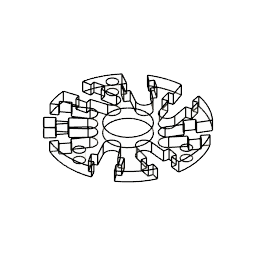
MidBearingMount-Mid_v21 (Autodesk Fusion 360 design; units mm, degrees)
Autodesk Fusion 360 part; units mm, degrees
other "Sketch1"
sketch "Sketch1" plane through (0, 0, 0) normal (0, 0, 1) x (1, 0, 0)
  circle A0 centre (0, 0) radius 20
  dimension "d1" = 40
  constraint coincident A0.centre origin
  measures "d1" diameter of A0
extrude "Extrude1" add sketch "Sketch1" along normal blind 3
sketch "sketch 220" plane through (0, 0, 0) normal (0, 0, 1) x (1, 0, 0)
  line L0 (55, -55) -> (-55, -55)
  line L1 (-55, -55) -> (-55, 55)
  line L2 (-55, 55) -> (55, 55)
  line L3 (55, 55) -> (55, -55)
  circle A0 centre (-27, 47) radius 3
  circle A1 centre (-1, 47) radius 3
  circle A2 centre (-47, -1) radius 3
  circle A3 centre (-47, -27) radius 3
  circle A4 centre (3.8268, 9.2388) radius 2.1
  line L4 (3.8268, 9.2388) -> (0, 0) construction
  circle A5 centre (-3.8268, 9.2388) radius 2.1
  circle A6 centre (-9.2388, 3.8268) radius 2.1
  circle A7 centre (-9.2388, -3.8268) radius 2.1
  circle A8 centre (-3.8268, -9.2388) radius 2.1
  circle A9 centre (3.8268, -9.2388) radius 2.1
  circle A10 centre (9.2388, -3.8268) radius 2.1
  circle A11 centre (9.2388, 3.8268) radius 2.1
  circle A12 centre (-47, -27) radius 3
  circle A13 centre (-47, -1) radius 3
  circle A14 centre (27, -47) radius 3
  circle A15 centre (1, -47) radius 3
  circle A16 centre (47, 27) radius 3
  circle A17 centre (47, 1) radius 3
  line L5 (3.8268, 9.2388) -> (-7.356, 51.4484) construction
  line L6 (-3.8267, 9.2387) -> (-39.1481, 32.3388) construction
  line L7 (-9.2241, 3.8302) -> (-38.1078, -2.8395) construction
  line L8 (-9.2387, -3.8268) -> (-45.7313, -32.4091) construction
  line L9 (-3.8418, -9.2572) -> (-24.5372, -34.632) construction
  line L10 (3.8268, -9.2388) -> (20.7131, -35.7055) construction
  line L11 (9.2388, -3.8268) -> (32.7897, -8.1449) construction
  line L12 (9.2388, 3.8268) -> (22.4195, 22.4675) construction
  line L13 (0, 0) -> (0, 3) construction
  line L14 (-38.1078, -2.8395) -> (1, -47) construction
  line L15 (32.7897, -8.1449) -> (27, -47) construction
  line L16 (20.7131, -35.7055) -> (47, 1) construction
  line L17 (-39.1481, 32.3388) -> (47, 27) construction
  line L18 (22.4195, 22.4675) -> (-1, 47) construction
  line L19 (-45.7313, -32.4091) -> (-27, 47) construction
  line L20 (-24.5372, -34.632) -> (-47, -27) construction
  line L21 (-7.356, 51.4484) -> (-47, -1) construction
  circle A18 centre (-26.9265, -6.4155) radius 6 construction
  circle A19 centre (-26.5529, -27.6103) radius 6 construction
  circle A20 centre (21, -25) radius 6 construction
  circle A21 centre (26, -13) radius 6 construction
  circle A22 centre (14.6683, 21.8979) radius 6 construction
  circle A23 centre (-10, 38) radius 6 construction
  circle A24 centre (-16.8843, 24.9475) radius 6 construction
  circle A25 centre (-35.9644, -17.138) radius 6 construction
  line L22 (-1.2763, 20.3008) -> (2.7836, 21.3764)
  line L23 (-1.2763, 20.3008) -> (1.7969, 8.701)
  line L24 (2.7836, 21.3764) -> (5.8568, 9.7766)
  line L25 (-15.0192, 14.0493) -> (-12.7204, 17.5644)
  line L26 (-20.4586, -0.9193) -> (-21.4036, 3.173)
  line L27 (-19.9809, -9.573) -> (-17.3911, -12.8795)
  line L28 (-13.0386, -17.2108) -> (-9.7838, -19.8654)
  line L29 (8.5109, -20.4847) -> (12.0516, -18.2256)
  line L30 (21.4208, -3.9254) -> (20.6633, -8.0565)
  line L31 (14.4523, 14.8373) -> (17.8816, 12.4124)
  line L32 (-12.7204, 17.5644) -> (-2.6774, 10.9963)
  line L33 (-15.0192, 14.0493) -> (-4.9762, 7.4813)
  line L34 (-21.4036, 3.173) -> (-9.7113, 5.873)
  line L35 (-20.4586, -0.9193) -> (-8.7663, 1.7807)
  line L36 (-19.9809, -9.573) -> (-10.5337, -2.1736)
  line L37 (-17.3911, -12.8795) -> (-7.9439, -5.4801)
  line L38 (-9.7838, -19.8654) -> (-2.1995, -10.5661)
  line L39 (-13.0386, -17.2108) -> (-5.4542, -7.9115)
  line L40 (12.0516, -18.2256) -> (5.5972, -8.1093)
  line L41 (8.5109, -20.4847) -> (2.0565, -10.3683)
  line L42 (20.6633, -8.0565) -> (8.8601, -5.8924)
  line L43 (21.4208, -3.9254) -> (9.6175, -1.7613)
  line L44 (14.4523, 14.8373) -> (7.5241, 5.0393)
  line L45 (17.8816, 12.4124) -> (10.9534, 2.6144)
  line L46 (26.6915, -34.8215) -> (30.8456, -35.4405)
  line L47 (-8.5279, -39.4086) -> (-5.3836, -36.6241)
  line L48 (-34.9623, -28.872) -> (-36.3135, -32.8488)
  line L49 (-41.4394, 9.8393) -> (-38.0888, 7.3067)
  line L50 (-31.7989, 35.8027) -> (-27.7111, 34.8384)
  line L51 (5.7671, 36.87) -> (8.8051, 39.7702)
  line L52 (35.1529, 29.8382) -> (34.8931, 25.6463)
  line L53 (38.3057, -7.5335) -> (41.7204, -9.9789)
  line L54 (30.8456, -35.4405) -> (29.9922, -47.2169)
  line L55 (26.6915, -34.8215) -> (24.0746, -46.3351)
  line L56 (-5.3836, -36.6241) -> (3.0893, -44.8472)
  line L57 (-8.5279, -39.4086) -> (-1.3897, -48.8137)
  line L58 (-34.9623, -28.872) -> (-45.8232, -24.2404)
  line L59 (-36.3135, -32.8488) -> (-47.7479, -29.9053)
  line L60 (-41.4394, 9.8393) -> (-49.2498, 0.9845)
  line L61 (-38.0888, 7.3067) -> (-44.477, -2.6231)
  line L62 (-27.7111, 34.8384) -> (-24.1405, 46.0928)
  line L63 (-31.7989, 35.8027) -> (-29.9635, 47.4663)
  line L64 (8.8051, 39.7702) -> (1.3202, 48.9018)
  line L65 (5.7671, 36.87) -> (-3.0074, 44.7706)
  line L66 (35.1529, 29.8382) -> (46.959, 29.9997)
  line L67 (34.8931, 25.6463) -> (46.5889, 24.0283)
  line L68 (41.7204, -9.9789) -> (49.3002, -0.9259)
  line L69 (38.3057, -7.5335) -> (44.436, 2.5576)
  circle A26 centre (-10, 38) radius 1.5
  circle A27 centre (-17, 25) radius 1.5
  circle A28 centre (14.6683, 21.8979) radius 1.5
  circle A29 centre (-26.9265, -6.4155) radius 1.5
  circle A30 centre (-36, -17) radius 1.5
  circle A31 centre (-26.5529, -27.6103) radius 1.5
  circle A32 centre (21, -25) radius 1.5
  circle A33 centre (26, -13) radius 1.5
  line L70 (-13.8698, 15.8068) -> (-3.8268, 9.2388) construction
  line L71 (0.7536, 20.8386) -> (3.8268, 9.2388) construction
  line L72 (9.2388, 3.8268) -> (16.1669, 13.6248) construction
  line L73 (9.2388, -3.8268) -> (21.042, -5.9909) construction
  line L74 (3.8268, -9.2388) -> (10.2813, -19.3551) construction
  line L75 (-3.8418, -9.2572) -> (-11.4112, -18.5381) construction
  line L76 (-9.2388, -3.8268) -> (-18.686, -11.2262) construction
  line L77 (-9.2241, 3.8302) -> (-20.9311, 1.1269) construction
  line L78 (-11.0342, 9.1729) -> (-6.6555, 15.8682) construction
  line L79 (-15.9776, 6.376) -> (-14.1776, -1.4189) construction
  line L80 (-16.4288, -4.3775) -> (-11.4959, -10.6756) construction
  line L81 (-10.7263, -11.3695) -> (-4.5268, -16.4258) construction
  line L82 (3.6819, -16.4484) -> (10.4262, -12.1455) construction
  line L83 (15.8618, -0.9745) -> (14.419, -8.8433) construction
  line L84 (9.4369, 11.0352) -> (15.9689, 6.4165) construction
  line L85 (-1.5764, 14.0143) -> (6.1568, 16.0631) construction
  line L86 (-7.9108, 16.6892) -> (-5.4001, 15.0472)
  line L87 (5.7727, 17.5131) -> (6.541, 14.6131)
  line L88 (-1.9605, 15.4643) -> (-1.1922, 12.5643)
  line L89 (-12.2895, 9.9939) -> (-9.7788, 8.3519)
  line L90 (-17.4391, 6.0385) -> (-14.516, 6.7135)
  line L91 (-15.6392, -1.7564) -> (-12.7161, -1.0814)
  line L92 (-17.6097, -5.3024) -> (-15.2479, -3.4525)
  line L93 (-12.6768, -11.6005) -> (-10.315, -9.7507)
  line L94 (-11.6743, -12.5319) -> (-9.7782, -10.2071)
  line L95 (-5.4748, -17.5882) -> (-3.5787, -15.2634)
  line L96 (2.8751, -15.1839) -> (4.4887, -17.713)
  line L97 (9.6194, -10.8809) -> (11.233, -13.41)
  line L98 (12.9436, -8.5728) -> (15.8945, -9.1138)
  line L99 (14.3864, -0.704) -> (17.3372, -1.245)
  line L100 (16.8349, 7.6412) -> (15.1028, 5.1917)
  line L101 (10.3029, 12.26) -> (8.5708, 9.8105)
  line L102 (5.7727, 17.5131) -> (3.9361, 17.0265)
  line L103 (6.541, 14.6131) -> (4.7044, 14.1265)
  line L104 (-1.9605, 15.4643) -> (-0.1239, 15.9509)
  line L105 (-1.1922, 12.5643) -> (0.6444, 13.0509)
  line L106 (-7.9108, 16.6892) -> (-8.8814, 15.0537)
  line L107 (-5.4001, 15.0472) -> (-6.4401, 13.4571)
  line L108 (-12.2895, 9.9939) -> (-11.2496, 11.584)
  line L109 (-9.7788, 8.3519) -> (-8.7389, 9.942)
  line L110 (-17.4391, 6.0385) -> (-17.0116, 4.1872)
  line L111 (-14.516, 6.7135) -> (-14.0886, 4.8622)
  line L112 (-12.7161, -1.0814) -> (-13.1436, 0.7699)
  line L113 (-15.6392, -1.7564) -> (-16.0666, 0.0949)
  line L114 (-15.2479, -3.4525) -> (-14.0764, -4.9483)
  line L115 (-17.6097, -5.3024) -> (-16.4382, -6.7982)
  line L116 (-10.315, -9.7507) -> (-11.4866, -8.2549)
  line L117 (-12.6768, -11.6005) -> (-13.8484, -10.1047)
  line L118 (-9.7782, -10.2071) -> (-8.3058, -11.408)
  line L119 (-11.6743, -12.5319) -> (-10.2019, -13.7328)
  line L120 (-3.5787, -15.2634) -> (-5.0511, -14.0625)
  line L121 (-5.4748, -17.5882) -> (-6.9472, -16.3873)
  line L122 (2.8751, -15.1839) -> (4.4769, -14.1619)
  line L123 (4.4887, -17.713) -> (6.0905, -16.691)
  line L124 (11.233, -13.41) -> (9.6312, -14.432)
  line L125 (9.6194, -10.8809) -> (8.0176, -11.9029)
  line L126 (15.8945, -9.1138) -> (16.2371, -7.245)
  line L127 (12.9436, -8.5728) -> (13.2863, -6.7039)
  line L128 (17.3372, -1.245) -> (16.9945, -3.1138)
  line L129 (14.3864, -0.704) -> (14.0437, -2.5728)
  line L130 (16.8349, 7.6412) -> (15.2835, 8.7382)
  line L131 (15.1028, 5.1917) -> (13.5515, 6.2887)
  line L132 (8.5708, 9.8105) -> (10.1222, 8.7135)
  line L133 (10.3029, 12.26) -> (11.8542, 11.163)
  line L134 (-6.9558, -38.0164) -> (1, -47) construction
  line L135 (27, -47) -> (28.7686, -35.131) construction
  line L136 (47, 1) -> (40.0131, -8.7562) construction
  line L137 (47, 27) -> (35.023, 27.7422) construction
  line L138 (-1, 47) -> (7.2861, 38.3201) construction
  line L139 (-27, 47) -> (-29.755, 35.3205) construction
  line L140 (-47, -1) -> (-39.7641, 8.573) construction
  line L141 (-47, -27) -> (-35.6379, -30.8604) construction
  line L142 (-6.7211, -45.8231) -> (0.7653, -39.1933) construction
  line L143 (22.9389, -40.3286) -> (32.8297, -41.8024) construction
  line L144 (39.4415, -0.9669) -> (47.5716, -6.7893) construction
  line L145 (41.3208, 32.3615) -> (40.7022, 22.3807) construction
  line L146 (-0.4736, 39.2075) -> (6.7597, 46.1126) construction
  line L147 (-33.2439, 42.3082) -> (-23.511, 40.0124) construction
  line L148 (-47.3708, 6.8014) -> (-39.3933, 0.7715) construction
  line L149 (-39.7105, -24.196) -> (-42.9275, -33.6644) construction
  line L150 (-7.7155, -44.7001) -> (-5.7266, -46.946)
  line L151 (-0.2292, -38.0703) -> (1.7598, -40.3162)
  line L152 (23.16, -38.845) -> (22.7178, -41.8122)
  line L153 (33.0508, -40.3188) -> (32.6086, -43.286)
  line L154 (38.5681, -2.1864) -> (40.3148, 0.2527)
  line L155 (46.6982, -8.0088) -> (48.445, -5.5698)
  line L156 (39.2051, 22.4735) -> (42.1994, 22.2879)
  line L157 (39.8236, 32.4543) -> (42.8179, 32.2688)
  line L158 (-1.5093, 40.2925) -> (0.5622, 38.1225)
  line L159 (5.7239, 47.1976) -> (7.7954, 45.0276)
  line L160 (-32.8996, 43.7681) -> (-33.5883, 40.8482)
  line L161 (-23.8554, 38.5524) -> (-23.1667, 41.4723)
  line L162 (-48.2753, 5.6048) -> (-46.4663, 7.9981)
  line L163 (-40.2978, -0.4251) -> (-38.4888, 1.9682)
  line L164 (-41.1307, -23.7134) -> (-38.2902, -24.6785)
  line L165 (-44.3477, -33.1819) -> (-41.5072, -34.147)
  line L166 (-7.7155, -44.7001) -> (-5.7996, -43.0034)
  line L167 (-5.7266, -46.946) -> (-3.9807, -45.3999)
  line L168 (-0.2292, -38.0703) -> (-2.1451, -39.7671)
  line L169 (1.7598, -40.3162) -> (0.0138, -41.8624)
  line L170 (23.16, -38.845) -> (25.6913, -39.2222)
  line L171 (22.7178, -41.8122) -> (25.0245, -42.156)
  line L172 (33.0508, -40.3188) -> (30.5194, -39.9416)
  line L173 (32.6086, -43.286) -> (30.3019, -42.9423)
  line L174 (40.3148, 0.2527) -> (42.2109, -1.1052)
  line L175 (38.5681, -2.1864) -> (40.6488, -3.6765)
  line L176 (48.445, -5.5698) -> (46.5489, -4.2119)
  line L177 (46.6982, -8.0088) -> (44.6175, -6.5187)
  line L178 (39.8236, 32.4543) -> (39.6653, 29.8999)
  line L179 (42.8179, 32.2688) -> (42.6736, 29.9411)
  line L180 (42.1994, 22.2879) -> (42.3436, 24.6156)
  line L181 (39.2051, 22.4735) -> (39.3634, 25.0279)
  line L182 (-1.5093, 40.2925) -> (0.1776, 41.9029)
  line L183 (0.5622, 38.1225) -> (2.4134, 39.8897)
  line L184 (7.7954, 45.0276) -> (5.9442, 43.2604)
  line L185 (5.7239, 47.1976) -> (4.037, 45.5872)
  line L186 (-32.8996, 43.7681) -> (-30.6297, 43.2327)
  line L187 (-33.5883, 40.8482) -> (-31.0974, 40.2607)
  line L188 (-23.1667, 41.4723) -> (-25.4365, 42.0077)
  line L189 (-23.8554, 38.5524) -> (-26.3463, 39.14)
  line L190 (-46.4663, 7.9981) -> (-44.4246, 6.4548)
  line L191 (-48.2753, 5.6048) -> (-46.4148, 4.1986)
  line L192 (-38.4888, 1.9682) -> (-40.5305, 3.5114)
  line L193 (-40.2978, -0.4251) -> (-42.1583, 0.9812)
  line L194 (-38.2902, -24.6785) -> (-39.1135, -27.1018)
  line L195 (-41.1307, -23.7134) -> (-41.881, -25.9216)
  line L196 (-41.5072, -34.147) -> (-40.6839, -31.7237)
  line L197 (-44.3477, -33.1819) -> (-43.5975, -30.9737)
  line L198 (1, -47) -> (27, -47) construction
  line L199 (-47, -1) -> (-47, -27) construction
  line L200 (47, 1) -> (47, 27) construction
  line L201 (-1, 47) -> (-27, 47) construction
  circle A34 centre (14, -47) radius 1.5
  circle A35 centre (-47, -14) radius 1.5
  circle A36 centre (47, 14) radius 1.5
  circle A37 centre (-14, 47) radius 1.5
  circle A38 centre (0, 0) radius 6
  line L202 (-15.5118, 13.2961) -> (-12.2278, 18.3176)
  line L203 (-21.6061, 4.0499) -> (-20.2561, -1.7962)
  line L204 (-20.5358, -8.8644) -> (-16.8361, -13.588)
  line L205 (-13.736, -16.642) -> (-9.0864, -20.4342)
  line L206 (7.7522, -20.9687) -> (12.8103, -17.7415)
  line L207 (20.501, -8.9418) -> (21.5831, -3.0401)
  line L208 (13.7174, 15.3569) -> (18.6164, 11.8928)
  line L209 (-2.1463, 20.0703) -> (3.6536, 21.6069)
  line L210 (1.7969, 8.701) -> (-2.1463, 20.0703)
  line L211 (3.6536, 21.6069) -> (5.8568, 9.7766)
  line L212 (13.7174, 15.3569) -> (7.4388, 4.9085)
  line L213 (18.6164, 11.8928) -> (10.9534, 2.6144)
  line L214 (21.5831, -3.0401) -> (9.6175, -1.7613)
  line L215 (20.501, -8.9418) -> (8.8601, -5.8924)
  line L216 (12.8103, -17.7415) -> (5.5972, -8.1093)
  line L217 (7.7522, -20.9687) -> (2.0565, -10.3683)
  line L218 (-13.736, -16.642) -> (-5.4542, -7.9115)
  line L219 (-9.0864, -20.4342) -> (-2.1995, -10.5661)
  line L220 (-20.5358, -8.8644) -> (-10.5337, -2.1736)
  line L221 (-16.8361, -13.588) -> (-7.9439, -5.4801)
  line L222 (-21.6061, 4.0499) -> (-9.7113, 5.873)
  line L223 (-20.2561, -1.7962) -> (-8.6156, 1.8214)
  line L224 (-15.5118, 13.2961) -> (-4.8425, 7.4007)
  line L225 (-12.2278, 18.3176) -> (-2.6774, 10.9963)
  point P0 (0.7536, 20.8386)
  point P1 (-13.8698, 15.8068)
  point P2 (-20.9311, 1.1269)
  point P3 (-18.686, -11.2262)
  point P4 (-11.4112, -18.5381)
  point P5 (10.2813, -19.3551)
  point P6 (21.042, -5.9909)
  point P7 (16.1669, 13.6248)
  point P8 (28.7686, -35.131)
  point P9 (-6.9558, -38.0164)
  point P10 (-35.6379, -30.8604)
  point P11 (-39.7641, 8.573)
  point P12 (-29.755, 35.3205)
  point P13 (7.2861, 38.3201)
  point P14 (35.023, 27.7422)
  point P15 (40.0131, -8.7562)
  point P16 (-8.8448, 12.5205)
  point P17 (-15.0776, 2.4786)
  point P18 (-13.9624, -7.5265)
  point P19 (-7.6265, -13.8976)
  point P20 (7.054, -14.297)
  point P21 (15.1404, -4.9089)
  point P22 (12.7029, 8.7258)
  point P23 (2.2902, 15.0387)
  point P24 (-2.9779, -42.5082)
  point P25 (27.8843, -41.0655)
  point P26 (43.5065, -3.8781)
  point P27 (41.0115, 27.3711)
  point P28 (3.1431, 42.6601)
  point P29 (-28.3775, 41.1603)
  point P30 (-43.3821, 3.7865)
  point P31 (-41.319, -28.9302)
extrude "Extrude2" cut sketch "sketch 220" along normal blind 12 contours A4 | A4 L22 L23 L24 L209 | L24 L103 L211 | L23 L105 L210 | L24 L102 L103 L211 | L87 L102 L103 L211 | L23 L104 L105 L210 | L88 L104 L105 L210 | L24 L102 L209 L211 | L23 L104 L209 L210 | A5 | A5 L25 L32 L33 L202 | L32 L107 L225 | A5 L33 L109 L224 | L32 L106 L107 L225 | L86 L106 L107 L225 | L33 L108 L109 L224 | L89 L108 L109 L224 | L32 L106 L202 L225 | L33 L108 L202 L224 | A6 | A6 L26 L34 L35 L203 | L34 L111 L222 | A6 L35 L112 L223 | L34 L110 L111 L222 | L90 L110 L111 L222 | L35 L112 L113 L223 | L91 L112 L113 L223 | L34 L110 L203 L222 | L35 L113 L203 L223 | A7 | A7 L27 L36 L37 L204 | L36 L114 L220 | L37 L116 L221 | L36 L114 L115 L220 | L92 L114 L115 L220 | L37 L116 L117 L221 | L93 L116 L117 L221 | L36 L115 L204 L220 | L37 L117 L204 L221 | A8 | A8 L28 L38 L39 L205 | L39 L118 L218 | L38 L120 L219 | L39 L118 L119 L218 | L94 L118 L119 L218 | L38 L120 L121 L219 | L95 L120 L121 L219 | L39 L119 L205 L218 | L38 L121 L205 L219 | A9 | A9 L29 L40 L41 L206 | L40 L125 L216 | L41 L122 L217 | L40 L124 L125 L216 | L97 L124 L125 L216 | L41 L122 L123 L217 | L96 L122 L123 L217 | L40 L124 L206 L216 | L41 L123 L206 L217 | A10 | A10 L30 L42 L43 L207 | L43 L129 L214 | L42 L127 L215 | L43 L128 L129 L214 | L99 L128 L129 L214 | L42 L126 L127 L215 | L98 L126 L127 L215 | L43 L128 L207 L214 | L42 L126 L207 L215 | A11 | A11 L31 L44 L45 L208 | A11 L44 L132 L212 | L45 L131 L213 | L44 L132 L133 L212 | L45 L130 L131 L213 | L100 L130 L131 L213 | L101 L132 L133 L212 | L44 L133 L208 L212 | L45 L130 L208 L213
extrude "Extrude3" cut sketch "sketch 220" along normal blind 5 contours A38
sketch "Sketch3" plane through (0, 0, 3) normal (0, 0, 1) x (-1, 0, 0)
  circle A0 centre (0, 0) radius 6
  arc A1 (2.0842, -19.8911) -> (10.5209, -17.0091) centre (0, 0) ccw
  line L0 (8.5964, -15.5338) -> (7.9108, -16.6892)
  line L1 (7.9108, -16.6892) -> (5.4001, -15.0472)
  line L2 (5.4001, -15.0472) -> (6.2555, -13.7393)
  arc A2 (4.8425, -7.4007) -> (2.6774, -10.9963) centre (3.8268, -9.2388) ccw
  line L3 (8.9254, -9.6568) -> (9.7788, -8.3519)
  line L4 (9.7788, -8.3519) -> (12.2895, -9.9939)
  line L5 (12.2895, -9.9939) -> (11.5585, -11.1117)
  line L6 (17.1381, -4.7347) -> (17.4391, -6.0385)
  line L7 (17.4391, -6.0385) -> (14.516, -6.7135)
  line L8 (14.516, -6.7135) -> (14.1644, -5.1905)
  arc A3 (8.6156, -1.8214) -> (9.7113, -5.873) centre (9.2388, -3.8268) ccw
  line L9 (13.0669, -0.438) -> (12.7161, 1.0814)
  line L10 (12.7161, 1.0814) -> (15.6392, 1.7564)
  line L11 (15.6392, 1.7564) -> (15.9397, 0.4548)
  line L12 (16.785, 6.3554) -> (17.6097, 5.3024)
  line L13 (17.6097, 5.3024) -> (15.2479, 3.4525)
  line L14 (15.2479, 3.4525) -> (14.2845, 4.6826)
  arc A4 (7.9439, 5.4801) -> (10.5337, 2.1736) centre (9.2388, 3.8268) ccw
  line L15 (11.2785, 8.5206) -> (10.315, 9.7507)
  line L16 (10.315, 9.7507) -> (12.6768, 11.6005)
  line L17 (12.6768, 11.6005) -> (13.5015, 10.5475)
  line L18 (10.6385, 13.3767) -> (11.6743, 12.5319)
  line L19 (11.6743, 12.5319) -> (9.7782, 10.2071)
  line L20 (9.7782, 10.2071) -> (8.5681, 11.1941)
  arc A5 (2.1995, 10.5661) -> (5.4542, 7.9115) centre (3.8268, 9.2388) ccw
  line L21 (4.7889, 14.2764) -> (3.5787, 15.2634)
  line L22 (3.5787, 15.2634) -> (5.4748, 17.5882)
  line L23 (5.4748, 17.5882) -> (6.5106, 16.7434)
  line L24 (-5.6163, 16.9936) -> (-4.4887, 17.713)
  line L25 (-4.4887, 17.713) -> (-2.8751, 15.1839)
  line L26 (-2.8751, 15.1839) -> (-4.1924, 14.3435)
  arc A6 (-5.5972, 8.1093) -> (-2.0565, 10.3683) centre (-3.8268, 9.2388) ccw
  line L27 (-8.3021, 11.7214) -> (-9.6194, 10.8809)
  line L28 (-9.6194, 10.8809) -> (-11.233, 13.41)
  line L29 (-11.233, 13.41) -> (-10.1054, 14.1294)
  line L30 (-16.1357, 7.7982) -> (-15.8945, 9.1138)
  line L31 (-15.8945, 9.1138) -> (-12.9436, 8.5728)
  line L32 (-12.9436, 8.5728) -> (-13.2254, 7.0359)
  arc A7 (-9.6175, 1.7613) -> (-8.8601, 5.8924) centre (-9.2388, 3.8268) ccw
  line L33 (-14.1046, 2.2408) -> (-14.3864, 0.704)
  line L34 (-14.3864, 0.704) -> (-17.3372, 1.245)
  line L35 (-17.3372, 1.245) -> (-17.096, 2.5606)
  line L36 (-15.7428, -8.4134) -> (-16.8349, -7.6412)
  line L37 (-16.8349, -7.6412) -> (-15.1028, -5.1917)
  line L38 (-15.1028, -5.1917) -> (-13.8271, -6.0938)
  arc A8 (-7.4388, -4.9085) -> (-10.9534, -2.6144) centre (-9.2388, -3.8268) ccw
  line L39 (-9.8436, -8.9105) -> (-8.5708, -9.8105)
  line L40 (-8.5708, -9.8105) -> (-10.3029, -12.26)
  line L41 (-10.3029, -12.26) -> (-11.3932, -11.489)
  line L42 (-4.4798, -17.1705) -> (-5.7727, -17.5131)
  line L43 (-5.7727, -17.5131) -> (-6.541, -14.6131)
  line L44 (-6.541, -14.6131) -> (-5.0306, -14.213)
  arc A9 (-1.7969, -8.701) -> (-5.8568, -9.7766) centre (-3.8268, -9.2388) ccw
  line L45 (-0.3182, -12.9645) -> (1.1922, -12.5643)
  line L46 (1.1922, -12.5643) -> (1.9605, -15.4643)
  line L47 (1.9605, -15.4643) -> (0.6676, -15.8068)
  circle A10 centre (0, 0) radius 6
  line L48 (-4.4769, 14.1619) -> (-2.0565, 10.3683)
  line L49 (12.0317, 15.9762) -> (5.4542, 7.9115)
  arc A11 (8.3893, 18.1554) -> (-7.317, 18.6135) centre (0, 0) ccw
  arc A12 (-5.5972, 8.1093) -> (-2.0565, 10.3683) centre (-3.8268, 9.2388) ccw
  line L50 (7.9439, 5.4801) -> (16.0987, 11.8672)
  arc A13 (-1.7969, -8.701) -> (-5.8568, -9.7766) centre (-3.8268, -9.2388) ccw
  arc A14 (-19.6724, 3.6048) -> (-16.7895, -10.868) centre (0, 0) ccw
  arc A15 (8.3893, 18.1554) -> (-7.317, 18.6135) centre (0, 0) ccw
  circle A16 centre (0, 0) radius 6
  line L51 (-3.2173, -19.7395) -> (-3.9361, -17.0265)
  line L52 (-4.4887, 17.713) -> (-2.8751, 15.1839)
  line L53 (-16.2371, 7.245) -> (-15.8945, 9.1138)
  line L54 (8.3058, 11.408) -> (5.4542, 7.9115)
  line L55 (18.2381, 8.208) -> (16.4382, 6.7982)
  line L56 (-13.5515, -6.2887) -> (-10.9534, -2.6144)
  arc A17 (8.7663, -1.7807) -> (9.7113, -5.873) centre (9.2388, -3.8268) ccw
  line L57 (-12.9436, 8.5728) -> (-13.2863, 6.7039)
  line L58 (-7.317, 18.6135) -> (-2.0565, 10.3683)
  line L59 (-8.5708, -9.8105) -> (-10.3029, -12.26)
  line L60 (-7.5241, -5.0393) -> (-10.1222, -8.7135)
  line L61 (16.0666, -0.0949) -> (19.9836, 0.8096)
  line L62 (15.6392, 1.7564) -> (16.0666, -0.0949)
  line L63 (-7.317, 18.6135) -> (-6.0905, 16.691)
  arc A18 (-9.6175, 1.7613) -> (-8.8601, 5.8924) centre (-9.2388, 3.8268) ccw
  line L64 (-9.6312, 14.432) -> (-11.0565, 16.6659)
  arc A19 (-5.5972, 8.1093) -> (-2.0565, 10.3683) centre (-3.8268, 9.2388) ccw
  line L65 (-5.5972, 8.1093) -> (-8.0176, 11.9029)
  line L66 (-17.3372, 1.245) -> (-16.9945, 3.1138)
  line L67 (11.4866, 8.2549) -> (10.315, 9.7507)
  line L68 (10.315, 9.7507) -> (12.6768, 11.6005)
  line L69 (4.9762, -7.4813) -> (14.5381, -13.7347)
  line L70 (9.7782, 10.2071) -> (8.3058, 11.408)
  line L71 (4.9762, -7.4813) -> (8.7389, -9.942)
  line L72 (9.7788, -8.3519) -> (12.2895, -9.9939)
  line L73 (16.4382, 6.7982) -> (17.6097, 5.3024)
  line L74 (13.8484, 10.1047) -> (16.0987, 11.8672)
  line L75 (-7.5241, -5.0393) -> (-14.0355, -14.2479)
  line L76 (5.4001, -15.0472) -> (6.4401, -13.4571)
  line L77 (17.6097, 5.3024) -> (15.2479, 3.4525)
  arc A20 (-11.0565, 16.6659) -> (-18.4768, 7.6556) centre (0, 0) ccw
  arc A21 (2.1995, 10.5661) -> (5.4542, 7.9115) centre (3.8268, 9.2388) ccw
  line L78 (17.4391, -6.0385) -> (14.516, -6.7135)
  line L79 (-9.6175, 1.7613) -> (-19.6724, 3.6048)
  line L80 (19.6785, -3.5714) -> (17.0116, -4.1872)
  line L81 (12.6768, 11.6005) -> (13.8484, 10.1047)
  line L82 (12.0317, 15.9762) -> (10.2019, 13.7328)
  line L83 (1.9605, -15.4643) -> (0.1239, -15.9509)
  line L84 (6.9472, 16.3873) -> (8.3893, 18.1554)
  line L85 (7.9439, 5.4801) -> (11.4866, 8.2549)
  arc A22 (7.9439, 5.4801) -> (10.5337, 2.1736) centre (9.2388, 3.8268) ccw
  line L86 (14.0886, -4.8622) -> (9.7113, -5.873)
  line L87 (15.2479, 3.4525) -> (14.0764, 4.9483)
  arc A23 (1.1873, -19.9647) -> (11.1999, -16.5699) centre (0, 0) ccw
  line L88 (5.0511, 14.0625) -> (3.5787, 15.2634)
  line L89 (-11.8542, -11.163) -> (-14.0355, -14.2479)
  arc A24 (7.9439, 5.4801) -> (10.5337, 2.1736) centre (9.2388, 3.8268) ccw
  line L90 (-3.2173, -19.7395) -> (-5.8568, -9.7766)
  line L91 (-16.7895, -10.868) -> (-15.2835, -8.7382)
  arc A25 (19.9836, 0.8096) -> (18.2381, 8.208) centre (0, 0) ccw
  arc A26 (-14.0355, -14.2479) -> (-3.2173, -19.7395) centre (0, 0) ccw
  line L92 (-5.5972, 8.1093) -> (-11.0565, 16.6659)
  line L93 (-10.1222, -8.7135) -> (-8.5708, -9.8105)
  line L94 (11.1999, -16.5699) -> (2.6774, -10.9963)
  arc A27 (8.7663, -1.7807) -> (9.7113, -5.873) centre (9.2388, -3.8268) ccw
  line L95 (-4.7044, -14.1265) -> (-5.8568, -9.7766)
  arc A28 (2.1995, 10.5661) -> (5.4542, 7.9115) centre (3.8268, 9.2388) ccw
  line L96 (-5.7727, -17.5131) -> (-6.541, -14.6131)
  line L97 (-3.9361, -17.0265) -> (-5.7727, -17.5131)
  line L98 (-10.3029, -12.26) -> (-11.8542, -11.163)
  line L99 (-16.8349, -7.6412) -> (-15.1028, -5.1917)
  line L100 (-15.1028, -5.1917) -> (-13.5515, -6.2887)
  arc A29 (-19.6724, 3.6048) -> (-16.7895, -10.868) centre (0, 0) ccw
  line L101 (-15.2835, -8.7382) -> (-16.8349, -7.6412)
  arc A30 (-7.5241, -5.0393) -> (-10.9534, -2.6144) centre (-9.2388, -3.8268) ccw
  arc A31 (-14.0355, -14.2479) -> (-3.2173, -19.7395) centre (0, 0) ccw
  arc A32 (-1.7969, -8.701) -> (-5.8568, -9.7766) centre (-3.8268, -9.2388) ccw
  line L102 (8.7663, -1.7807) -> (19.9836, 0.8096)
  arc A33 (16.0987, 11.8672) -> (12.0317, 15.9762) centre (0, 0) ccw
  line L103 (-14.0437, 2.5728) -> (-14.3864, 0.704)
  arc A34 (4.9762, -7.4813) -> (2.6774, -10.9963) centre (3.8268, -9.2388) ccw
  line L104 (-1.7969, -8.701) -> (1.1873, -19.9647)
  circle A35 centre (-17, -2.5) radius 1.5
  line L105 (18.2381, 8.208) -> (10.5337, 2.1736)
  arc A36 (1.1873, -19.9647) -> (11.1999, -16.5699) centre (0, 0) ccw
  arc A37 (-11.0565, 16.6659) -> (-18.4768, 7.6556) centre (0, 0) ccw
  line L106 (-6.541, -14.6131) -> (-4.7044, -14.1265)
  arc A38 (-7.5241, -5.0393) -> (-10.9534, -2.6144) centre (-9.2388, -3.8268) ccw
  arc A39 (14.5381, -13.7347) -> (19.6785, -3.5714) centre (0, 0) ccw
  line L107 (10.2019, 13.7328) -> (11.6743, 12.5319)
  line L108 (0.1239, -15.9509) -> (1.1873, -19.9647)
  arc A40 (14.5381, -13.7347) -> (19.6785, -3.5714) centre (0, 0) ccw
  line L109 (8.7389, -9.942) -> (9.7788, -8.3519)
  circle A41 centre (14.4882, -9.2272) radius 1.5
  line L110 (14.516, -6.7135) -> (14.0886, -4.8622)
  line L111 (12.2895, -9.9939) -> (11.2496, -11.584)
  line L112 (1.1922, -12.5643) -> (1.9605, -15.4643)
  line L113 (5.4748, 17.5882) -> (6.9472, 16.3873)
  line L114 (11.2496, -11.584) -> (14.5381, -13.7347)
  line L115 (-0.6444, -13.0509) -> (1.1922, -12.5643)
  circle A42 centre (0.3491, 15.9537) radius 1.5
  line L116 (13.1436, -0.7699) -> (12.7161, 1.0814)
  line L117 (7.9108, -16.6892) -> (5.4001, -15.0472)
  arc A43 (19.9836, 0.8096) -> (18.2381, 8.208) centre (0, 0) ccw
  line L118 (-1.7969, -8.701) -> (-0.6444, -13.0509)
  line L119 (11.1999, -16.5699) -> (8.8814, -15.0537)
  line L120 (17.0116, -4.1872) -> (17.4391, -6.0385)
  line L121 (2.1995, 10.5661) -> (8.3893, 18.1554)
  line L122 (8.8814, -15.0537) -> (7.9108, -16.6892)
  line L123 (6.4401, -13.4571) -> (2.6774, -10.9963)
  arc A44 (4.9762, -7.4813) -> (2.6774, -10.9963) centre (3.8268, -9.2388) ccw
  line L124 (-11.233, 13.41) -> (-9.6312, 14.432)
  line L125 (-16.9945, 3.1138) -> (-19.6724, 3.6048)
  line L126 (8.7663, -1.7807) -> (13.1436, -0.7699)
  line L127 (-16.7895, -10.868) -> (-10.9534, -2.6144)
  line L128 (-2.8751, 15.1839) -> (-4.4769, 14.1619)
  arc A45 (16.0987, 11.8672) -> (12.0317, 15.9762) centre (0, 0) ccw
  line L129 (-8.0176, 11.9029) -> (-9.6194, 10.8809)
  line L130 (11.6743, 12.5319) -> (9.7782, 10.2071)
  line L131 (-6.0905, 16.691) -> (-4.4887, 17.713)
  line L132 (-15.8945, 9.1138) -> (-12.9436, 8.5728)
  line L133 (-18.4768, 7.6556) -> (-8.8601, 5.8924)
  arc A46 (-9.6175, 1.7613) -> (-8.8601, 5.8924) centre (-9.2388, 3.8268) ccw
  line L134 (-18.4768, 7.6556) -> (-16.2371, 7.245)
  line L135 (-13.2863, 6.7039) -> (-8.8601, 5.8924)
  line L136 (14.0764, 4.9483) -> (10.5337, 2.1736)
  line L137 (3.5787, 15.2634) -> (5.4748, 17.5882)
  line L138 (-9.6175, 1.7613) -> (-14.0437, 2.5728)
  line L139 (19.6785, -3.5714) -> (9.7113, -5.873)
  line L140 (-14.3864, 0.704) -> (-17.3372, 1.245)
  line L141 (2.1995, 10.5661) -> (5.0511, 14.0625)
  line L142 (-9.6194, 10.8809) -> (-11.233, 13.41)
  line L143 (12.7161, 1.0814) -> (15.6392, 1.7564)
  line L144 (0.6676, -15.8068) -> (2.0842, -19.8911)
  line L145 (10.5209, -17.0091) -> (8.5964, -15.5338)
  line L146 (6.2555, -13.7393) -> (2.6774, -10.9963)
  line L147 (4.8425, -7.4007) -> (8.9254, -9.6568)
  line L148 (11.5585, -11.1117) -> (15.1269, -13.0834)
  arc A47 (15.1269, -13.0834) -> (19.5167, -4.3702) centre (0, 0) ccw
  line L149 (19.5167, -4.3702) -> (17.1381, -4.7347)
  line L150 (14.1644, -5.1905) -> (9.7113, -5.873)
  line L151 (8.6156, -1.8214) -> (13.0669, -0.438)
  line L152 (15.9397, 0.4548) -> (19.9281, 1.6943)
  arc A48 (19.9281, 1.6943) -> (18.531, 7.5233) centre (0, 0) ccw
  line L153 (18.531, 7.5233) -> (16.785, 6.3554)
  line L154 (14.2845, 4.6826) -> (10.5337, 2.1736)
  line L155 (7.9439, 5.4801) -> (11.2785, 8.5206)
  line L156 (13.5015, 10.5475) -> (15.6253, 12.484)
  arc A49 (15.6253, 12.484) -> (12.6468, 15.4938) centre (0, 0) ccw
  line L157 (12.6468, 15.4938) -> (10.6385, 13.3767)
  line L158 (8.5681, 11.1941) -> (5.4542, 7.9115)
  line L159 (2.1995, 10.5661) -> (4.7889, 14.2764)
  line L160 (6.5106, 16.7434) -> (7.7058, 18.4559)
  arc A50 (7.7058, 18.4559) -> (-6.625, 18.8709) centre (0, 0) ccw
  line L161 (-6.625, 18.8709) -> (-5.6163, 16.9936)
  line L162 (-4.1924, 14.3435) -> (-2.0565, 10.3683)
  line L163 (-5.5972, 8.1093) -> (-8.3021, 11.7214)
  line L164 (-10.1054, 14.1294) -> (-11.6815, 16.234)
  arc A51 (-11.6815, 16.234) -> (-18.1809, 8.334) centre (0, 0) ccw
  line L165 (-18.1809, 8.334) -> (-16.1357, 7.7982)
  line L166 (-13.2254, 7.0359) -> (-8.8601, 5.8924)
  line L167 (-9.6175, 1.7613) -> (-14.1046, 2.2408)
  line L168 (-17.096, 2.5606) -> (-19.796, 2.8491)
  arc A52 (-19.796, 2.8491) -> (-17.2097, -10.1895) centre (0, 0) ccw
  line L169 (-17.2097, -10.1895) -> (-15.7428, -8.4134)
  line L170 (-13.8271, -6.0938) -> (-10.9534, -2.6144)
  line L171 (-7.4388, -4.9085) -> (-9.8436, -8.9105)
  line L172 (-11.3932, -11.489) -> (-13.4072, -14.8407)
  arc A53 (-13.4072, -14.8407) -> (-4.0292, -19.5899) centre (0, 0) ccw
  line L173 (-4.0292, -19.5899) -> (-4.4798, -17.1705)
  line L174 (-5.0306, -14.213) -> (-5.8568, -9.7766)
  line L175 (-1.7969, -8.701) -> (-0.3182, -12.9645)
  dimension "d17" = 3
  dimension "d18" = 3
  dimension "d19" = 3
  measures "d17" diameter of A35
  measures "d18" diameter of A41
  measures "d19" diameter of A42
extrude "Extrude5" cut sketch "Sketch3" against normal blind 9 contours A35 | A41 | A42
sketch "LaserMidBearingMountMid-Bearing" plane through (0, 0, 3) normal (0, 0, 1) x (-1, 0, 0)
  circle A0 centre (14.4882, -9.2272) radius 1.5
  circle A1 centre (-17, -2.5) radius 1.5
  circle A2 centre (0.3491, 15.9537) radius 1.5
  circle A3 centre (0, 0) radius 6
  line L0 (0.6676, -15.8068) -> (2.0842, -19.8911)
  arc A4 (2.0842, -19.8911) -> (10.5209, -17.0091) centre (0, 0) ccw
  line L1 (10.5209, -17.0091) -> (8.5964, -15.5338)
  line L2 (8.5964, -15.5338) -> (7.9108, -16.6892)
  line L3 (7.9108, -16.6892) -> (5.4001, -15.0472)
  line L4 (5.4001, -15.0472) -> (6.2555, -13.7393)
  line L5 (6.2555, -13.7393) -> (2.6774, -10.9963)
  arc A5 (4.8425, -7.4007) -> (2.6774, -10.9963) centre (3.8268, -9.2388) ccw
  line L6 (4.8425, -7.4007) -> (8.9254, -9.6568)
  line L7 (8.9254, -9.6568) -> (9.7788, -8.3519)
  line L8 (9.7788, -8.3519) -> (12.2895, -9.9939)
  line L9 (12.2895, -9.9939) -> (11.5585, -11.1117)
  line L10 (11.5585, -11.1117) -> (15.1269, -13.0834)
  arc A6 (15.1269, -13.0834) -> (19.5167, -4.3702) centre (0, 0) ccw
  line L11 (19.5167, -4.3702) -> (17.1381, -4.7347)
  line L12 (17.1381, -4.7347) -> (17.4391, -6.0385)
  line L13 (17.4391, -6.0385) -> (14.516, -6.7135)
  line L14 (14.516, -6.7135) -> (14.1644, -5.1905)
  line L15 (14.1644, -5.1905) -> (9.7113, -5.873)
  arc A7 (8.6156, -1.8214) -> (9.7113, -5.873) centre (9.2388, -3.8268) ccw
  line L16 (8.6156, -1.8214) -> (13.0669, -0.438)
  line L17 (13.0669, -0.438) -> (12.7161, 1.0814)
  line L18 (12.7161, 1.0814) -> (15.6392, 1.7564)
  line L19 (15.6392, 1.7564) -> (15.9397, 0.4548)
  line L20 (15.9397, 0.4548) -> (19.9281, 1.6943)
  arc A8 (19.9281, 1.6943) -> (18.531, 7.5233) centre (0, 0) ccw
  line L21 (18.531, 7.5233) -> (16.785, 6.3554)
  line L22 (16.785, 6.3554) -> (17.6097, 5.3024)
  line L23 (17.6097, 5.3024) -> (15.2479, 3.4525)
  line L24 (15.2479, 3.4525) -> (14.2845, 4.6826)
  line L25 (14.2845, 4.6826) -> (10.5337, 2.1736)
  arc A9 (7.9439, 5.4801) -> (10.5337, 2.1736) centre (9.2388, 3.8268) ccw
  line L26 (7.9439, 5.4801) -> (11.2785, 8.5206)
  line L27 (11.2785, 8.5206) -> (10.315, 9.7507)
  line L28 (10.315, 9.7507) -> (12.6768, 11.6005)
  line L29 (12.6768, 11.6005) -> (13.5015, 10.5475)
  line L30 (13.5015, 10.5475) -> (15.6253, 12.484)
  arc A10 (15.6253, 12.484) -> (12.6468, 15.4938) centre (0, 0) ccw
  line L31 (12.6468, 15.4938) -> (10.6385, 13.3767)
  line L32 (10.6385, 13.3767) -> (11.6743, 12.5319)
  line L33 (11.6743, 12.5319) -> (9.7782, 10.2071)
  line L34 (9.7782, 10.2071) -> (8.5681, 11.1941)
  line L35 (8.5681, 11.1941) -> (5.4542, 7.9115)
  arc A11 (2.1995, 10.5661) -> (5.4542, 7.9115) centre (3.8268, 9.2388) ccw
  line L36 (2.1995, 10.5661) -> (4.7889, 14.2764)
  line L37 (4.7889, 14.2764) -> (3.5787, 15.2634)
  line L38 (3.5787, 15.2634) -> (5.4748, 17.5882)
  line L39 (5.4748, 17.5882) -> (6.5106, 16.7434)
  line L40 (6.5106, 16.7434) -> (7.7058, 18.4559)
  arc A12 (7.7058, 18.4559) -> (-6.625, 18.8709) centre (0, 0) ccw
  line L41 (-6.625, 18.8709) -> (-5.6163, 16.9936)
  line L42 (-5.6163, 16.9936) -> (-4.4887, 17.713)
  line L43 (-4.4887, 17.713) -> (-2.8751, 15.1839)
  line L44 (-2.8751, 15.1839) -> (-4.1924, 14.3435)
  line L45 (-4.1924, 14.3435) -> (-2.0565, 10.3683)
  arc A13 (-5.5972, 8.1093) -> (-2.0565, 10.3683) centre (-3.8268, 9.2388) ccw
  line L46 (-5.5972, 8.1093) -> (-8.3021, 11.7214)
  line L47 (-8.3021, 11.7214) -> (-9.6194, 10.8809)
  line L48 (-9.6194, 10.8809) -> (-11.233, 13.41)
  line L49 (-11.233, 13.41) -> (-10.1054, 14.1294)
  line L50 (-10.1054, 14.1294) -> (-11.6815, 16.234)
  arc A14 (-11.6815, 16.234) -> (-18.1809, 8.334) centre (0, 0) ccw
  line L51 (-18.1809, 8.334) -> (-16.1357, 7.7982)
  line L52 (-16.1357, 7.7982) -> (-15.8945, 9.1138)
  line L53 (-15.8945, 9.1138) -> (-12.9436, 8.5728)
  line L54 (-12.9436, 8.5728) -> (-13.2254, 7.0359)
  line L55 (-13.2254, 7.0359) -> (-8.8601, 5.8924)
  arc A15 (-9.6175, 1.7613) -> (-8.8601, 5.8924) centre (-9.2388, 3.8268) ccw
  line L56 (-9.6175, 1.7613) -> (-14.1046, 2.2408)
  line L57 (-14.1046, 2.2408) -> (-14.3864, 0.704)
  line L58 (-14.3864, 0.704) -> (-17.3372, 1.245)
  line L59 (-17.3372, 1.245) -> (-17.096, 2.5606)
  line L60 (-17.096, 2.5606) -> (-19.796, 2.8491)
  arc A16 (-19.796, 2.8491) -> (-17.2097, -10.1895) centre (0, 0) ccw
  line L61 (-17.2097, -10.1895) -> (-15.7428, -8.4134)
  line L62 (-15.7428, -8.4134) -> (-16.8349, -7.6412)
  line L63 (-16.8349, -7.6412) -> (-15.1028, -5.1917)
  line L64 (-15.1028, -5.1917) -> (-13.8271, -6.0938)
  line L65 (-13.8271, -6.0938) -> (-10.9534, -2.6144)
  arc A17 (-7.4388, -4.9085) -> (-10.9534, -2.6144) centre (-9.2388, -3.8268) ccw
  line L66 (-7.4388, -4.9085) -> (-9.8436, -8.9105)
  line L67 (-9.8436, -8.9105) -> (-8.5708, -9.8105)
  line L68 (-8.5708, -9.8105) -> (-10.3029, -12.26)
  line L69 (-10.3029, -12.26) -> (-11.3932, -11.489)
  line L70 (-11.3932, -11.489) -> (-13.4072, -14.8407)
  arc A18 (-13.4072, -14.8407) -> (-4.0292, -19.5899) centre (0, 0) ccw
  line L71 (-4.0292, -19.5899) -> (-4.4798, -17.1705)
  line L72 (-4.4798, -17.1705) -> (-5.7727, -17.5131)
  line L73 (-5.7727, -17.5131) -> (-6.541, -14.6131)
  line L74 (-6.541, -14.6131) -> (-5.0306, -14.213)
  line L75 (-5.0306, -14.213) -> (-5.8568, -9.7766)
  arc A19 (-1.7969, -8.701) -> (-5.8568, -9.7766) centre (-3.8268, -9.2388) ccw
  line L76 (-1.7969, -8.701) -> (-0.3182, -12.9645)
  line L77 (-0.3182, -12.9645) -> (1.1922, -12.5643)
  line L78 (1.1922, -12.5643) -> (1.9605, -15.4643)
  line L79 (1.9605, -15.4643) -> (0.6676, -15.8068)
